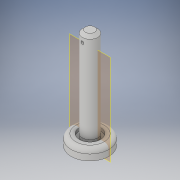
# Autodesk Inventor part: Fuß
Saved by Autodesk Inventor 2019 (Build 230136000, 136)
## iProperties
Created: 2018-07-23
Part Number: Fuß
Material: Generisch
Document SubType Name: Modeling
Designer: 1eule14
Density: 1 g/cm^3
Appearance: Vorgabe
Author: 1eule14
Autodesk Inventor part; units mm, degrees
ref_plane "YZ Plane" through (0, 0, 0) normal (1, 0, 0) x (0, 1, 0)
ref_plane "XZ Plane" through (0, 0, 0) normal (0, 1, 0) x (-1, 0, 0)
sketch "Skizze1" plane through (0, 0, 0) normal (0, 1, 0) x (-1, 0, 0)
  circle A0 centre (0, 0) radius 12.5
  dimension "d0" = 25
  constraints: 1 centre point, 1 coincident
  measures "d0" diameter of A0
extrude "Extrusion1" add sketch "Skizze1" along normal blind 7
fillet "Rundung1" radius 3 1 edges at (12.5, 7, 0)
sketch "Skizze2" plane through (0, 7, 0) normal (0, 1, 0) x (1, 0, 0)
  circle A0 centre (0, 0) radius 5.1
  dimension "d4" = 10.2
  constraints: 1 centre point, 1 coincident
  measures "d4" diameter of A0
extrude "Extrusion2" add sketch "Skizze2" along normal blind 60 separate body
ref_plane "Arbeitsebene1" through (0, 0, 0) normal (0, 0, 1) x (1, 0, 0)
sketch "Skizze3" plane through (0, 0, 0) normal (0, 0, 1) x (1, 0, 0)
  line L0 (5.1, 67) -> (-5.1, 67) projected
  line L1 (0, -11) -> (0, 66) projected
  point P0 (0, 0)
  point P1 (0, 62)
  point P2 (0, 62)
  dimension "d8" = 5
  constraints: 1 coincident, 1 point on line
  measures "d8" distance from line of L0 point (0, 62)
hole "Bohrung1" at (0, 62, 0) direction (0, 0, -1) diameter 2 end through all both bodies 2
chamfer "Fase1" distance 2 angle 45 1 edges at (-5.1, 67, 0)
sketch "Skizze4" plane through (0, 7, 0) normal (0, 1, 0) x (1, 0, 0)
  circle A0 centre (0, 0) radius 5.1 projected
  circle A1 centre (0, 0) radius 4.875
  line L0 (17.5, 0) -> (-17.5, 0) projected
  circle A2 centre (0, 0) radius 7
  dimension "d19" = 9.75
  dimension "d20" = 14
  constraints: 2 centre point, 1 coincident, 1 concentric, 1 midpoint
  measures "d19" diameter of A1
  measures "d20" diameter of A2
extrude "Extrusion3" cut sketch "Skizze4" against normal blind 2 contours L0 A2 A0 | A0 L0 A2 bodies 1
